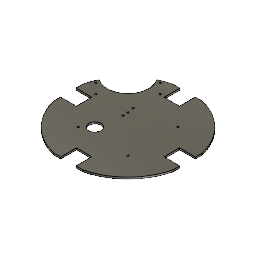
Rambots v6 (Autodesk Fusion 360 design; units mm, degrees)
Autodesk Fusion 360 part; units mm, degrees
sketch "Sketch2" plane through (0, 0, 0) normal (0, 0, 1) x (1, 0, 0) in component "Base plate"
  circle A0 centre (0, 0) radius 105
  line L0 (0, 0) -> (0, 105)
  line L1 (0, 0) -> (0, -105)
  line L2 (0, 0) -> (105, 0)
  line L3 (0, 0) -> (-105, 0)
  line L4 (-105, 0) -> (-102, 0)
  line L5 (-102, 0) -> (-102, 24.9199)
  line L6 (-102, 0) -> (-102, -24.9199)
  line L7 (-102, 24.9199) -> (-75, 24.9199)
  line L8 (-102, -24.9199) -> (-75, -24.9199)
  line L9 (-75, -24.9199) -> (-75, 24.9199)
  line L10 (0, 105) -> (0, 102)
  line L11 (0, 102) -> (24.9199, 102)
  line L12 (0, 102) -> (-24.9199, 102)
  line L13 (-24.9199, 102) -> (-24.9199, 75)
  line L14 (24.9199, 102) -> (24.9199, 75)
  line L15 (24.9199, 75) -> (-24.9199, 75)
  line L16 (105, 0) -> (102, 0)
  line L17 (102, 0) -> (102, 24.9199)
  line L18 (102, 0) -> (102, -24.9199)
  line L19 (102, -24.9199) -> (75, -24.9199)
  line L20 (102, 24.9199) -> (75, 24.9199)
  line L21 (75, 24.9199) -> (75, -24.9199)
  line L22 (0, -105) -> (0, -102)
  line L23 (0, -102) -> (24.9199, -102)
  line L24 (0, -102) -> (-24.9199, -102)
  line L25 (-24.9199, -102) -> (-24.9199, -75)
  line L26 (24.9199, -102) -> (24.9199, -75)
  line L27 (24.9199, -75) -> (-24.9199, -75)
  line L28 (0, 0) -> (3.7123, -3.7123)
  line L29 (0, 0) -> (5.25, 0) construction
  line L30 (0, 0) -> (-3.7123, 3.7123)
  line L31 (0, 0) -> (5.25, 0) construction
  line L32 (-3.7123, 3.7123) -> (-1.591, 5.8336)
  line L33 (-1.591, 5.8336) -> (8.909, 5.8336) construction
  line L34 (5.8336, -1.591) -> (3.7123, -3.7123)
  line L35 (3.7123, -3.7123) -> (1.591, -5.8336)
  line L36 (3.7123, -3.7123) -> (6.7123, -3.7123) construction
  line L37 (1.591, -5.8336) -> (12.091, -5.8336) construction
  line L38 (-5.8336, 1.591) -> (-3.7123, 3.7123)
  line L39 (-3.7123, 3.7123) -> (-1.591, 5.8336)
  line L40 (-75, 0) -> (-67.5, 0)
  line L41 (-67.5, 0) -> (-67.5, 13)
  line L42 (-67.5, 13) -> (-75, 13)
  line L43 (-75, 13) -> (-75, 0)
  line L44 (-67.5, 0) -> (-75, 0)
  line L45 (-75, 0) -> (-75, -13)
  line L46 (-75, -13) -> (-67.5, -13)
  line L47 (-67.5, -13) -> (-67.5, 0)
  line L48 (0, 75) -> (-13, 75)
  line L49 (-13, 75) -> (-13, 67.5)
  line L50 (-13, 67.5) -> (0, 67.5)
  line L51 (0, 67.5) -> (0, 75)
  line L52 (10, 75) -> (0, 75)
  line L53 (0, 75) -> (0, 67.5)
  line L54 (75, 0) -> (67.5, 0)
  line L55 (67.5, 0) -> (67.5, 13)
  line L56 (67.5, 13) -> (75, 13)
  line L57 (75, 13) -> (75, 0)
  line L58 (67.5, 0) -> (75, 0)
  line L59 (75, 0) -> (75, -10)
  line L60 (0, -75) -> (13, -75)
  line L61 (13, -75) -> (13, -67.5)
  line L62 (13, -67.5) -> (0, -67.5)
  line L63 (0, -67.5) -> (0, -75)
  line L64 (-10, -75) -> (0, -75)
  line L65 (0, -75) -> (0, -67.5)
  line L66 (0, -67.5) -> (-13, -67.5)
  line L67 (-13, -67.5) -> (-13, -75)
  line L68 (67.5, 0) -> (67.5, -13)
  line L69 (67.5, -13) -> (75, -13)
  line L70 (0, 67.5) -> (13, 67.5)
  line L71 (13, 67.5) -> (13, 75)
  line L72 (-13, 75) -> (-13, 102)
  line L73 (13, 75) -> (13, 102)
  line L74 (75, 13) -> (102, 13)
  line L75 (75, -13) -> (102, -13)
  line L76 (13, -75) -> (13, -102)
  line L77 (-13, -75) -> (-13, -102)
  line L78 (-75, -13) -> (-102, -13)
  line L79 (-75, 13) -> (-102, 13)
  dimension "d2" = 210
  dimension "d3" = 3
  dimension "d4" = 27
  dimension "d5" = 27
  dimension "d6" = 3
  dimension "d7" = 27
  dimension "d8" = 27
  dimension "d9" = 3
  dimension "d10" = 27
  dimension "d11" = 27
  dimension "d12" = 3
  dimension "d13" = 27
  dimension "d14" = 27
  dimension "d15" = 45
  dimension "d16" = 5.25
  dimension "d17" = 135
  dimension "d18" = 5.25
  dimension "d19" = 3
  dimension "d21" = 10.5
  dimension "d22" = 135
  dimension "d23" = 3
  dimension "d25" = 10.5
  dimension "d28" = 7.5
  dimension "d29" = 13
  dimension "d30" = 13
  dimension "d31" = 7.5
  dimension "d32" = 7.5
  dimension "d33" = 13
  dimension "d34" = 7.5
  dimension "d35" = 13
  dimension "d36" = 7.5
  dimension "d37" = 13
  dimension "d96" = 13
  dimension "d97" = 13
  dimension "d98" = 13
  dimension "d99" = 27
  constraint coincident A0.centre L0.start
  constraint coincident A0 L0.end
  constraint vertical L0
  constraint coincident A0 L1.end
  constraint parallel L0 L1
  constraint coincident A0 L2.end
  constraint perpendicular L1 L2
  constraint coincident A0 L3.end
  constraint perpendicular L1 L3
  constraint parallel L3 L4
  constraint vertical L5
  constraint coincident A0 L5.end
  constraint vertical L6
  constraint coincident A0 L6.end
  constraint perpendicular L5 L7
  constraint perpendicular L6 L8
  constraint parallel L0 L10
  constraint horizontal L11
  constraint coincident A0 L11.end
  constraint horizontal L12
  constraint coincident A0 L12.end
  constraint perpendicular L12 L13
  constraint perpendicular L11 L14
  constraint horizontal L16
  constraint vertical L17
  constraint coincident A0 L17.end
  constraint vertical L18
  constraint coincident A0 L18.end
  constraint perpendicular L18 L19
  constraint horizontal L20
  constraint perpendicular L19 L22
  constraint horizontal L23
  constraint coincident A0 L23.end
  constraint coincident A0 L24.end
  constraint perpendicular L1 L24
  constraint perpendicular L24 L25
  constraint vertical L26
  constraint horizontal L29
  constraint horizontal L31
  constraint perpendicular L30 L32
  constraint horizontal L33
  constraint horizontal L36
  constraint horizontal L37
  constraint horizontal L40
  constraint vertical L41
  constraint horizontal L42
  constraint vertical L43
  constraint midpoint L9 L40.start
  constraint horizontal L44
  constraint vertical L45
  constraint horizontal L46
  constraint vertical L47
  constraint horizontal L48
  constraint vertical L49
  constraint horizontal L50
  constraint vertical L51
  constraint midpoint L15 L48.start
  constraint horizontal L52
  constraint vertical L53
  constraint coincident L15 L52.start
  constraint horizontal L54
  constraint vertical L55
  constraint horizontal L56
  constraint vertical L57
  constraint midpoint L21 L54.start
  constraint horizontal L58
  constraint vertical L59
  constraint coincident L21 L59.end
  constraint horizontal L60
  constraint vertical L61
  constraint horizontal L62
  constraint vertical L63
  constraint midpoint L27 L60.start
  constraint horizontal L64
  constraint vertical L65
  constraint coincident L27 L64.start
  constraint perpendicular L1 L66
  constraint coincident L27 L67.end
  constraint perpendicular L27 L67
  constraint perpendicular L58 L68
  constraint coincident L21 L69.end
  constraint perpendicular L21 L69
  constraint perpendicular L51 L70
  constraint coincident L15 L71.end
  constraint perpendicular L15 L71
  constraint coincident L12 L72.end
  constraint perpendicular L12 L72
  constraint coincident L11 L73.end
  constraint perpendicular L11 L73
  constraint coincident L17 L74.end
  constraint perpendicular L17 L74
  constraint coincident L18 L75.end
  constraint perpendicular L18 L75
  constraint coincident L23 L76.end
  constraint perpendicular L23 L76
  constraint coincident L24 L77.end
  constraint perpendicular L24 L77
  constraint coincident L6 L78.end
  constraint perpendicular L6 L78
  constraint coincident L5 L79.end
  constraint perpendicular L5 L79
  measures "d2" diameter of A0
  measures "d3" distance of L3.end L4.end
  measures "d4" distance of L5.end L7.end
  measures "d5" distance of L6.end L8.end
  measures "d6" distance of L0.end L10.end
  measures "d7" distance of L12.end L13.end
  measures "d8" distance of L11.end L14.end
  measures "d9" distance of L2.end L16.end
  measures "d10" distance of L18.end L19.end
  measures "d11" distance of L17.end L20.end
  measures "d12" distance of L1.end L22.end
  measures "d13" distance of L24.end L25.end
  measures "d14" distance of L23.end L26.end
  measures "d15" angle of L28 L29
  measures "d16" distance of A0.centre L28.end
  measures "d17" angle of L30 L31
  measures "d18" distance of A0.centre L30.end
  measures "d19" distance of L30.end L32.end
  measures "d21" distance of L32.end L34.start
  measures "d22" angle of L35 L36
  measures "d23" distance of L28.end L35.end
  measures "d25" distance of L35.end L38.start
  measures "d28" distance of L40.start L40.end
  measures "d29" distance of L40.start L42.end
  measures "d30" distance of L40.end L46.end
  measures "d31" distance of L40.end L40.start
  measures "d32" distance of L48.start L50.end
  measures "d33" distance of L48.start L48.end
  measures "d34" distance of L54.start L54.end
  measures "d35" distance of L54.start L56.end
  measures "d36" distance of L60.start L62.end
  measures "d37" distance of L60.start L60.end
  measures "d96" distance of L62.end L66.end
  measures "d97" distance of L54.end L68.end
  measures "d98" distance of L50.end L70.end
  measures "d99" distance of L69.end L75.end
extrude "Extrude2" add sketch "Sketch2" along normal blind 3.175 contours A0 L0 L2 L14 L15 L20 L21 L55 L56 L70 L71 | L17 L20 L21 L74 | L18 L19 L21 L75 | A0 L1 L2 L19 L21 L26 L27 L61 L62 L68 L69 | L11 L14 L15 L73 | L23 L26 L27 L76 | L2 L21 L54 L58 L59 L68 L69 | L2 L21 L54 L55 L56 L57 L58 | A0 L0 L3 L7 L9 L13 L15 L41 L42 L49 L50 | L12 L13 L15 L72 | L0 L15 L51 L52 L53 L70 L71 | L24 L25 L27 L77 | A0 L1 L3 L8 L9 L25 L27 L46 L47 L66 L67 | L1 L27 L60 L61 L62 L63 L65 | L5 L7 L9 L79 | L0 L15 L48 L49 L50 L51 L53 | L6 L8 L9 L78 | L1 L27 L63 L64 L65 L66 L67 | L3 L9 L40 L44 L45 L46 L47 | L3 L9 L40 L41 L42 L43 L44 in component "Base plate"
sketch "Sketch3" plane through (0, 0, 0) normal (0, 0, -1) x (1, 0, 0) in component "Base plate"
  arc A0 (-102, -24.9199) -> (-24.9199, -102) centre (0, 0) ccw
  line L0 (13, 75) -> (-13, 75)
  line L1 (-75, 13) -> (-75, -13)
  line L2 (-13, -75) -> (13, -75)
  line L3 (75, -13) -> (75, 13)
  line L4 (-67.5, 0) -> (-65.5, 0)
  line L5 (-65.5, 0) -> (-24.25, 0)
  line L6 (-24.25, 0) -> (-24.25, 10)
  line L7 (-24.25, 10) -> (-65.5, 10)
  line L8 (-65.5, 10) -> (-65.5, 0)
  line L9 (-65.5, 0) -> (-24.25, 0)
  line L10 (-24.25, 0) -> (-24.25, -10)
  line L11 (-24.25, -10) -> (-65.5, -10)
  line L12 (-65.5, -10) -> (-65.5, 0)
  line L13 (-24.25, 0) -> (-11.25, 0)
  line L14 (-65.5, 0) -> (-59.5, 0)
  circle A1 centre (-59.5, 0) radius 1.5
  line L15 (-65.5, 10) -> (-57.75, 10)
  line L16 (-57.75, 10) -> (-56.25, 10)
  line L17 (-56.25, 10) -> (-56.25, 8)
  circle A2 centre (-56.25, 8) radius 1.5
  line L18 (-57.75, 10) -> (-57.75, 8)
  line L19 (-56.25, 10) -> (-54.75, 10)
  line L20 (-54.75, 10) -> (-54.75, 8)
  line L21 (-65.5, -10) -> (-57.75, -10)
  line L22 (-57.75, -10) -> (-56.25, -10)
  line L23 (-56.25, -10) -> (-54.75, -10)
  line L24 (-56.25, -10) -> (-56.25, -8)
  circle A3 centre (-56.25, -8) radius 1.5
  line L25 (-57.75, -10) -> (-57.75, -8)
  line L26 (-54.75, -10) -> (-54.75, -8)
  line L27 (-54.75, -10) -> (-32.4, -10)
  line L28 (-54.75, 10) -> (-32.4, 10)
  line L29 (-32.4, 10) -> (-30.9, 10)
  line L30 (-30.9, 10) -> (-29.4, 10)
  line L31 (-32.4, -10) -> (-30.9, -10)
  line L32 (-30.9, -10) -> (-29.4, -10)
  line L33 (-30.9, 10) -> (-30.9, 8)
  circle A4 centre (-30.9, 8) radius 1.5
  line L34 (-32.4, 10) -> (-32.4, 8)
  line L35 (-29.4, 10) -> (-29.4, 8)
  line L36 (-30.9, -10) -> (-30.9, -8)
  circle A5 centre (-30.9, -8) radius 1.5
  line L37 (-32.4, -10) -> (-32.4, -8)
  line L38 (-29.4, -10) -> (-29.4, -8)
  line L39 (2.1213, -2.1213) -> (14.4957, -14.4957)
  circle A6 centre (14.4957, -14.4957) radius 1.5
  line L40 (0, 0) -> (-74.2462, -74.2462)
  line L41 (-74.2462, -74.2462) -> (-56.5685, -56.5685)
  line L42 (0, 0) -> (-28.2843, 28.2843)
  line L43 (0, 0) -> (35, 0) construction
  circle A7 centre (-28.2843, 28.2843) radius 7.5
  line L44 (-102, 13) -> (-75, 13)
  line L45 (-75, -13) -> (-102, -13)
  line L46 (-102, -13) -> (-102, -24.9199)
  line L47 (-24.9199, -102) -> (-13, -102)
  line L48 (-13, -102) -> (-13, -75)
  line L49 (13, -75) -> (13, -102)
  line L50 (13, -102) -> (24.9199, -102)
  arc A8 (24.9199, -102) -> (102, -24.9199) centre (0, 0) ccw
  line L51 (102, -24.9199) -> (102, -13)
  line L52 (102, -13) -> (75, -13)
  line L53 (75, 13) -> (102, 13)
  line L54 (102, 13) -> (102, 24.9199)
  arc A9 (102, 24.9199) -> (24.9199, 102) centre (0, 0) ccw
  line L55 (24.9199, 102) -> (13, 102)
  line L56 (13, 102) -> (13, 75)
  line L57 (-13, 75) -> (-13, 102)
  line L58 (-13, 102) -> (-24.9199, 102)
  arc A10 (-24.9199, 102) -> (-102, 24.9199) centre (0, 0) ccw
  line L59 (-102, 24.9199) -> (-102, 13)
  circle A11 centre (-74.2462, -74.2462) radius 35
  line L60 (0, 0) -> (-21.2132, -21.2132)
  circle A12 centre (-21.2132, -21.2132) radius 1.5
  dimension "d40" = 2
  dimension "d41" = 41.25
  dimension "d42" = 10
  dimension "d43" = 10
  dimension "d44" = 41.25
  dimension "d45" = 13
  dimension "d46" = 6
  dimension "d47" = 3
  dimension "d48" = 7.75
  dimension "d49" = 1.5
  dimension "d50" = 3
  dimension "d51" = 1.5
  dimension "d52" = 7.75
  dimension "d53" = 1.5
  dimension "d54" = 1.5
  dimension "d55" = 2
  dimension "d56" = 3
  dimension "d57" = 22.35
  dimension "d58" = 22.35
  dimension "d59" = 1.5
  dimension "d60" = 1.5
  dimension "d61" = 1.5
  dimension "d62" = 1.5
  dimension "d63" = 2
  dimension "d64" = 3
  dimension "d65" = 2
  dimension "d66" = 3
  dimension "d67" = 2
  dimension "d72" = 17.5
  dimension "d73" = 3
  dimension "d77" = 25
  dimension "d90" = 135
  dimension "d91" = 40
  dimension "d93" = 15
  dimension "d105" = 70
  dimension "d106" = 30
  dimension "d107" = 3
  constraint horizontal L4
  constraint horizontal L5
  constraint vertical L6
  constraint horizontal L7
  constraint vertical L8
  constraint horizontal L9
  constraint vertical L10
  constraint horizontal L11
  constraint vertical L12
  constraint perpendicular L6 L13
  constraint perpendicular L8 L14
  constraint coincident L14.end A1.centre
  constraint perpendicular L8 L15
  constraint parallel L7 L16
  constraint perpendicular L16 L17
  constraint coincident L17.end A2.centre
  constraint coincident A2 L18.end
  constraint tangent A2 L18
  constraint perpendicular L7 L18
  constraint perpendicular L18 L19
  constraint coincident A2 L20.end
  constraint tangent A2 L20
  constraint perpendicular L19 L20
  constraint perpendicular L12 L21
  constraint parallel L11 L22
  constraint parallel L11 L23
  constraint perpendicular L23 L24
  constraint coincident L24.end A3.centre
  constraint coincident A3 L25.end
  constraint tangent A3 L25
  constraint coincident A3 L26.end
  constraint tangent A3 L26
  constraint perpendicular L26 L27
  constraint perpendicular L20 L28
  constraint parallel L7 L29
  constraint parallel L7 L30
  constraint parallel L11 L31
  constraint parallel L11 L32
  constraint perpendicular L29 L33
  constraint coincident L33.end A4.centre
  constraint coincident A4 L34.end
  constraint tangent A4 L34
  constraint coincident A4 L35.end
  constraint tangent A4 L35
  constraint perpendicular L32 L36
  constraint coincident L36.end A5.centre
  constraint coincident A5 L37.end
  constraint tangent A5 L37
  constraint coincident A5 L38.end
  constraint tangent A5 L38
  constraint coincident L39.end A6.centre
  constraint coincident A0.centre L40.start
  constraint parallel L40 L41
  constraint horizontal L43
  constraint coincident L42.end A7.centre
  constraint coincident L40.end L41.start
  constraint perpendicular L42 L60
  constraint coincident L60.end A12.centre
  measures "d40" distance of L4.start L4.end
  measures "d41" distance of L4.end L5.end
  measures "d42" distance of L4.end L7.end
  measures "d43" distance of L4.end L11.end
  measures "d44" distance of L4.end L5.end
  measures "d45" distance of L5.end L13.end
  measures "d46" distance of L4.end L14.end
  measures "d47" diameter of A1
  measures "d48" distance of L7.end L15.end
  measures "d49" distance of L15.end L16.end
  measures "d50" diameter of A2
  measures "d51" distance of L16.end L19.end
  measures "d52" distance of L11.end L21.end
  measures "d53" distance of L21.end L22.end
  measures "d54" distance of L22.end L23.end
  measures "d55" distance of L22.end L24.end
  measures "d56" diameter of A3
  measures "d57" distance of L23.end L27.end
  measures "d58" distance of L19.end L28.end
  measures "d59" distance of L28.end L29.end
  measures "d60" distance of L29.end L30.end
  measures "d61" distance of L27.end L31.end
  measures "d62" distance of L31.end L32.end
  measures "d63" distance of L29.end L33.end
  measures "d64" diameter of A4
  measures "d65" distance of L31.end L36.end
  measures "d66" diameter of A5
  measures "d67" distance of L16.end L17.end
  measures "d72" distance of L39.start L39.end
  measures "d73" diameter of A6
  measures "d77" distance of L40.end L41.end
  measures "d90" angle of L42 L43
  measures "d91" distance of A0.centre L42.end
  measures "d93" diameter of A7
  measures "d105" diameter of A11
  measures "d106" distance of A0.centre L60.end
  measures "d107" diameter of A12
sketch "Sketch1" plane through (0, 0, 0) normal (1, 0, 0) x (0, 1, 0) in component "Base plate"
  line L0 (-5.8336, 3.175) -> (1.591, 3.175)
  line L1 (0, 10) -> (0, -5)
  constraint perpendicular L0 L1
extrude "Extrude3" cut sketch "Sketch3" against normal blind 20 contours A0 L40 L41 A11 | A0 L40 L41 A11 in component "Base plate"
sketch "Sketch2 (1)" plane through (0, 0, 3.175) normal (0, 0, 1) x (-1, 0, 0) in component "Base plate"
  line L0 (75, -13) -> (75, 13)
  line L1 (13, 75) -> (-13, 75)
  arc A0 (94.524, -45.7188) -> (102, -24.9199) centre (0, 0) ccw
  line L2 (-75, 13) -> (-75, -13)
  line L3 (-13, -75) -> (13, -75)
  line L4 (0, 0) -> (-42.4264, -42.4264)
  line L5 (0, 0) -> (65, 0) construction
  line L6 (-15.5563, -15.5563) -> (-33.9411, -33.9411)
  circle A1 centre (-42.4264, -42.4264) radius 1.5
  line L7 (102, -24.9199) -> (102, -13)
  line L8 (102, -13) -> (75, -13)
  line L9 (75, 13) -> (102, 13)
  line L10 (102, 13) -> (102, 24.9199)
  arc A2 (102, 24.9199) -> (24.9199, 102) centre (0, 0) ccw
  line L11 (24.9199, 102) -> (13, 102)
  line L12 (13, 102) -> (13, 75)
  line L13 (-13, 75) -> (-13, 102)
  line L14 (-13, 102) -> (-24.9199, 102)
  arc A3 (-24.9199, 102) -> (-102, 24.9199) centre (0, 0) ccw
  line L15 (-102, 24.9199) -> (-102, 13)
  line L16 (-102, 13) -> (-75, 13)
  line L17 (-75, -13) -> (-102, -13)
  line L18 (-102, -13) -> (-102, -24.9199)
  arc A4 (-102, -24.9199) -> (-24.9199, -102) centre (0, 0) ccw
  line L19 (-24.9199, -102) -> (-13, -102)
  line L20 (-13, -102) -> (-13, -75)
  line L21 (13, -75) -> (13, -102)
  line L22 (13, -102) -> (24.9199, -102)
  arc A5 (24.9199, -102) -> (45.7188, -94.524) centre (0, 0) ccw
  arc A6 (94.524, -45.7188) -> (45.7188, -94.524) centre (74.2462, -74.2462) ccw
  dimension "d82" = 135
  dimension "d83" = 60
  dimension "d84" = 26
  dimension "d85" = 3
  constraint horizontal L5
  constraint coincident A0.centre L4.start
  constraint coincident L4 L6.start
  constraint parallel L4 L6
  constraint coincident L4.end A1.centre
  measures "d82" angle of L4 L5
  measures "d83" distance of A0.centre L4.end
  measures "d84" distance of L6.start L6.end
  measures "d85" diameter of A1
extrude "Extrude4" cut sketch "Sketch2 (1)" against normal blind 10 contours A1 in component "Base plate"
pattern_circular "C-Pattern2" count 4 over 360 about axis through (0, 0, 1.75) along (0, 0, 1) of 1 faces at (43.8086, 41.8438, 2.1167) in component "Base plate"
extrude "Extrude5" cut sketch "Sketch3" against normal blind 20 contours A7 in component "Base plate"
sketch "Sketch4" plane through (0, 0, 0) normal (1, 0, 0) x (0, 1, 0)
sketch "Sketch5" plane through (0, 0, 3.175) normal (0, 0, 1) x (-1, 0, 0)
  circle A0 centre (28.2843, 28.2843) radius 7.5
  circle A1 centre (-42.4264, 42.4264) radius 1.5
  circle A2 centre (42.4264, 42.4264) radius 1.5
  circle A3 centre (42.4264, -42.4264) radius 1.5
  circle A4 centre (-42.4264, -42.4264) radius 1.5
  arc A5 (94.524, -45.7188) -> (102, -24.9199) centre (0, 0) ccw
  line L0 (102, -24.9199) -> (102, -13)
  line L1 (102, -13) -> (75, -13)
  line L2 (75, -13) -> (75, 13)
  line L3 (75, 13) -> (102, 13)
  line L4 (102, 13) -> (102, 24.9199)
  arc A6 (102, 24.9199) -> (24.9199, 102) centre (0, 0) ccw
  line L5 (24.9199, 102) -> (13, 102)
  line L6 (13, 102) -> (13, 75)
  line L7 (13, 75) -> (-13, 75)
  line L8 (-13, 75) -> (-13, 102)
  line L9 (-13, 102) -> (-24.9199, 102)
  arc A7 (-24.9199, 102) -> (-102, 24.9199) centre (0, 0) ccw
  line L10 (-102, 24.9199) -> (-102, 13)
  line L11 (-102, 13) -> (-75, 13)
  line L12 (-75, 13) -> (-75, -13)
  line L13 (-75, -13) -> (-102, -13)
  line L14 (-102, -13) -> (-102, -24.9199)
  arc A8 (-102, -24.9199) -> (-24.9199, -102) centre (0, 0) ccw
  line L15 (-24.9199, -102) -> (-13, -102)
  line L16 (-13, -102) -> (-13, -75)
  line L17 (-13, -75) -> (13, -75)
  line L18 (13, -75) -> (13, -102)
  line L19 (13, -102) -> (24.9199, -102)
  arc A9 (24.9199, -102) -> (45.7188, -94.524) centre (0, 0) ccw
  line L20 (0, 0) -> (-21.2132, -21.2132)
  line L21 (0, 0) -> (30, 0) construction
  circle A10 centre (-21.2132, -21.2132) radius 1.5
  arc A11 (94.524, -45.7188) -> (45.7188, -94.524) centre (74.2462, -74.2462) ccw
  dimension "d100" = 135
  dimension "d101" = 30
  dimension "d102" = 3
  constraint horizontal L21
  constraint coincident A5.centre A6.centre
  constraint coincident L20.end A10.centre
  measures "d100" angle of L20 L21
  measures "d101" distance of A5.centre L20.end
  measures "d102" diameter of A10
extrude "Extrude6" cut sketch "Sketch5" against normal blind 35 contours A10 in component "Base plate"
extrude "Extrude7" cut sketch "Sketch3" against normal blind 6 contours L40 L60 A12 | L40 L60 A12 in component "Base plate"
sketch "Sketch6" plane through (0, 0, 3.175) normal (0, 0, 1) x (-1, 0, 0)
  circle A0 centre (21.2132, -21.2132) radius 1.5
  circle A1 centre (-21.2132, -21.2132) radius 1.5
  circle A2 centre (28.2843, 28.2843) radius 7.5
  circle A3 centre (-42.4264, 42.4264) radius 1.5
  circle A4 centre (42.4264, 42.4264) radius 1.5
  circle A5 centre (42.4264, -42.4264) radius 1.5
  circle A6 centre (-42.4264, -42.4264) radius 1.5
  arc A7 (94.524, -45.7188) -> (45.7188, -94.524) centre (74.2462, -74.2462) ccw
  arc A8 (94.524, -45.7188) -> (102, -24.9199) centre (0, 0) ccw
  line L0 (102, -24.9199) -> (102, -13)
  line L1 (102, -13) -> (75, -13)
  line L2 (75, -13) -> (75, 13)
  line L3 (75, 13) -> (102, 13)
  line L4 (102, 13) -> (102, 24.9199)
  arc A9 (102, 24.9199) -> (24.9199, 102) centre (0, 0) ccw
  line L5 (24.9199, 102) -> (13, 102)
  line L6 (13, 102) -> (13, 75)
  line L7 (13, 75) -> (-13, 75)
  line L8 (-13, 75) -> (-13, 102)
  line L9 (-13, 102) -> (-24.9199, 102)
  arc A10 (-24.9199, 102) -> (-102, 24.9199) centre (0, 0) ccw
  line L10 (-102, 24.9199) -> (-102, 13)
  line L11 (-102, 13) -> (-75, 13)
  line L12 (-75, 13) -> (-75, -13)
  line L13 (-75, -13) -> (-102, -13)
  line L14 (-102, -13) -> (-102, -24.9199)
  arc A11 (-102, -24.9199) -> (-24.9199, -102) centre (0, 0) ccw
  line L15 (-24.9199, -102) -> (-13, -102)
  line L16 (-13, -102) -> (-13, -75)
  line L17 (-13, -75) -> (13, -75)
  line L18 (13, -75) -> (13, -102)
  line L19 (13, -102) -> (24.9199, -102)
  arc A12 (24.9199, -102) -> (45.7188, -94.524) centre (0, 0) ccw
  circle A13 centre (42.4264, -42.4264) radius 1.5
  constraint concentric A5 A13
extrude "Extrude8" add sketch "Sketch6" against normal blind 3.175 contours A5 A13 in component "Base plate"
sketch "Sketch7" plane through (0, 0, 3.175) normal (0, 0, 1) x (-1, 0, 0)
  circle A0 centre (21.2132, -21.2132) radius 1.5
  circle A1 centre (-21.2132, -21.2132) radius 1.5
  circle A2 centre (28.2843, 28.2843) radius 7.5
  circle A3 centre (-42.4264, 42.4264) radius 1.5
  circle A4 centre (42.4264, 42.4264) radius 1.5
  circle A5 centre (-42.4264, -42.4264) radius 1.5
  arc A6 (94.524, -45.7188) -> (45.7188, -94.524) centre (74.2462, -74.2462) ccw
  arc A7 (94.524, -45.7188) -> (102, -24.9199) centre (0, 0) ccw
  line L0 (102, -24.9199) -> (102, -13)
  line L1 (102, -13) -> (75, -13)
  line L2 (75, -13) -> (75, 13)
  line L3 (75, 13) -> (102, 13)
  line L4 (102, 13) -> (102, 24.9199)
  arc A8 (102, 24.9199) -> (24.9199, 102) centre (0, 0) ccw
  line L5 (24.9199, 102) -> (13, 102)
  line L6 (13, 102) -> (13, 75)
  line L7 (13, 75) -> (-13, 75)
  line L8 (-13, 75) -> (-13, 102)
  line L9 (-13, 102) -> (-24.9199, 102)
  arc A9 (-24.9199, 102) -> (-102, 24.9199) centre (0, 0) ccw
  line L10 (-102, 24.9199) -> (-102, 13)
  line L11 (-102, 13) -> (-75, 13)
  line L12 (-75, 13) -> (-75, -13)
  line L13 (-75, -13) -> (-102, -13)
  line L14 (-102, -13) -> (-102, -24.9199)
  arc A10 (-102, -24.9199) -> (-24.9199, -102) centre (0, 0) ccw
  line L15 (-24.9199, -102) -> (-13, -102)
  line L16 (-13, -102) -> (-13, -75)
  line L17 (-13, -75) -> (13, -75)
  line L18 (13, -75) -> (13, -102)
  line L19 (13, -102) -> (24.9199, -102)
  arc A11 (24.9199, -102) -> (45.7188, -94.524) centre (0, 0) ccw
  circle A12 centre (28.2843, 28.2843) radius 10.5
  dimension "d112" = 21
  constraint concentric A2 A12
  measures "d112" diameter of A12
extrude "Extrude9" cut sketch "Sketch7" against normal blind 20 contours A12 in component "Base plate"
sketch "Sketch8" plane through (0, 0, 3.175) normal (0, 0, 1) x (-1, 0, 0)
  circle A0 centre (28.2843, 28.2843) radius 10.5
  circle A1 centre (21.2132, -21.2132) radius 1.5
  circle A2 centre (-21.2132, -21.2132) radius 1.5
  circle A3 centre (-42.4264, 42.4264) radius 1.5
  circle A4 centre (42.4264, 42.4264) radius 1.5
  circle A5 centre (-42.4264, -42.4264) radius 1.5
  arc A6 (94.524, -45.7188) -> (45.7188, -94.524) centre (74.2462, -74.2462) ccw
  arc A7 (94.524, -45.7188) -> (102, -24.9199) centre (0, 0) ccw
  line L0 (102, -24.9199) -> (102, -13)
  line L1 (102, -13) -> (75, -13)
  line L2 (75, -13) -> (75, 13)
  line L3 (75, 13) -> (102, 13)
  line L4 (102, 13) -> (102, 24.9199)
  arc A8 (102, 24.9199) -> (24.9199, 102) centre (0, 0) ccw
  line L5 (24.9199, 102) -> (13, 102)
  line L6 (13, 102) -> (13, 75)
  line L7 (13, 75) -> (-13, 75)
  line L8 (-13, 75) -> (-13, 102)
  line L9 (-13, 102) -> (-24.9199, 102)
  arc A9 (-24.9199, 102) -> (-102, 24.9199) centre (0, 0) ccw
  line L10 (-102, 24.9199) -> (-102, 13)
  line L11 (-102, 13) -> (-75, 13)
  line L12 (-75, 13) -> (-75, -13)
  line L13 (-75, -13) -> (-102, -13)
  line L14 (-102, -13) -> (-102, -24.9199)
  arc A10 (-102, -24.9199) -> (-24.9199, -102) centre (0, 0) ccw
  line L15 (-24.9199, -102) -> (-13, -102)
  line L16 (-13, -102) -> (-13, -75)
  line L17 (-13, -75) -> (13, -75)
  line L18 (13, -75) -> (13, -102)
  line L19 (13, -102) -> (24.9199, -102)
  arc A11 (24.9199, -102) -> (45.7188, -94.524) centre (0, 0) ccw
  circle A12 centre (-21.2132, -21.2132) radius 1.5
  constraint concentric A2 A12
extrude "Extrude10" add sketch "Sketch8" against normal blind 3.175 contours A2 A12 in component "Base plate"
sketch "Sketch9" plane through (0, 0, 0) normal (0, 0, -1) x (1, 0, 0)
  circle A0 centre (-28.2843, 28.2843) radius 10.5
  circle A1 centre (-21.2132, -21.2132) radius 1.5
  circle A2 centre (42.4264, 42.4264) radius 1.5
  circle A3 centre (-42.4264, 42.4264) radius 1.5
  circle A4 centre (42.4264, -42.4264) radius 1.5
  arc A5 (-45.7188, -94.524) -> (-94.524, -45.7188) centre (-74.2462, -74.2462) ccw
  arc A6 (-45.7188, -94.524) -> (-24.9199, -102) centre (0, 0) ccw
  line L0 (-24.9199, -102) -> (-13, -102)
  line L1 (-13, -102) -> (-13, -75)
  line L2 (-13, -75) -> (13, -75)
  line L3 (13, -75) -> (13, -102)
  line L4 (13, -102) -> (24.9199, -102)
  arc A7 (24.9199, -102) -> (102, -24.9199) centre (0, 0) ccw
  line L5 (102, -24.9199) -> (102, -13)
  line L6 (102, -13) -> (75, -13)
  line L7 (75, -13) -> (75, 13)
  line L8 (75, 13) -> (102, 13)
  line L9 (102, 13) -> (102, 24.9199)
  arc A8 (102, 24.9199) -> (24.9199, 102) centre (0, 0) ccw
  line L10 (24.9199, 102) -> (13, 102)
  line L11 (13, 102) -> (13, 75)
  line L12 (13, 75) -> (-13, 75)
  line L13 (-13, 75) -> (-13, 102)
  line L14 (-13, 102) -> (-24.9199, 102)
  arc A9 (-24.9199, 102) -> (-102, 24.9199) centre (0, 0) ccw
  line L15 (-102, 24.9199) -> (-102, 13)
  line L16 (-102, 13) -> (-75, 13)
  line L17 (-75, 13) -> (-75, -13)
  line L18 (-75, -13) -> (-102, -13)
  line L19 (-102, -13) -> (-102, -24.9199)
  arc A10 (-102, -24.9199) -> (-94.524, -45.7188) centre (0, 0) ccw
  line L20 (13, -75) -> (-75, 13)
  line L21 (-31, -31) -> (-23.2218, -38.7782)
  line L22 (-31, -31) -> (-38.7782, -23.2218)
  line L23 (-38.7782, -23.2218) -> (-35.2426, -19.6863)
  line L24 (-35.2426, -19.6863) -> (-19.6863, -35.2426)
  line L25 (-19.6863, -35.2426) -> (-23.2218, -38.7782)
  line L26 (-27.4645, -27.4645) -> (-23.2218, -31.7071)
  line L27 (-27.4645, -27.4645) -> (-31.7071, -23.2218)
  circle A11 centre (-23.2218, -31.7071) radius 1.5
  line L28 (-23.2218, -31.7071) -> (-12.6152, -21.1005)
  line L29 (-12.6152, -21.1005) -> (-21.1005, -12.6152)
  circle A12 centre (-21.1005, -12.6152) radius 1.5
  dimension "d117" = 11
  dimension "d118" = 11
  dimension "d119" = 5
  dimension "d120" = 22
  dimension "d121" = 6
  dimension "d122" = 6
  dimension "d123" = 3
  dimension "d124" = 15
  dimension "d125" = 12
  dimension "d126" = 3
  constraint coincident L2.end L3.start
  constraint coincident L16.end L17.start
  constraint midpoint L20 L21.start
  constraint parallel L20 L21
  constraint parallel L20 L22
  constraint perpendicular L22 L23
  constraint perpendicular L23 L24
  constraint midpoint L24 L26.start
  constraint perpendicular L25 L26
  constraint parallel L24 L27
  constraint coincident L26.end A11.centre
  constraint perpendicular L24 L28
  constraint perpendicular L28 L29
  constraint coincident L29.end A12.centre
  measures "d117" distance of L21.start L21.end
  measures "d118" distance of L21.start L22.end
  measures "d119" distance of L22.end L23.end
  measures "d120" distance of L23.end L24.end
  measures "d121" distance of L26.start L26.end
  measures "d122" distance of L26.start L27.end
  measures "d123" diameter of A11
  measures "d124" distance of L26.end L28.end
  measures "d125" distance of L28.end L29.end
  measures "d126" diameter of A12
extrude "Extrude11" cut sketch "Sketch9" against normal blind 16 contours L24 L26 A11 | L24 A11 L28 | L24 L26 A11 L28 | A12 in component "Base plate"
sketch "Sketch10" plane through (0, 0, 0) normal (0, 0, -1) x (1, 0, 0)
  circle A0 centre (-23.2218, -31.7071) radius 1.5
  circle A1 centre (-21.1005, -12.6152) radius 1.5
  circle A2 centre (-28.2843, 28.2843) radius 10.5
  circle A3 centre (-21.2132, -21.2132) radius 1.5
  circle A4 centre (42.4264, 42.4264) radius 1.5
  circle A5 centre (-42.4264, 42.4264) radius 1.5
  circle A6 centre (42.4264, -42.4264) radius 1.5
  arc A7 (-45.7188, -94.524) -> (-94.524, -45.7188) centre (-74.2462, -74.2462) ccw
  arc A8 (-45.7188, -94.524) -> (-24.9199, -102) centre (0, 0) ccw
  line L0 (-24.9199, -102) -> (-13, -102)
  line L1 (-13, -102) -> (-13, -75)
  line L2 (-13, -75) -> (13, -75)
  line L3 (13, -75) -> (13, -102)
  line L4 (13, -102) -> (24.9199, -102)
  arc A9 (24.9199, -102) -> (102, -24.9199) centre (0, 0) ccw
  line L5 (102, -24.9199) -> (102, -13)
  line L6 (102, -13) -> (75, -13)
  line L7 (75, -13) -> (75, 13)
  line L8 (75, 13) -> (102, 13)
  line L9 (102, 13) -> (102, 24.9199)
  arc A10 (102, 24.9199) -> (24.9199, 102) centre (0, 0) ccw
  line L10 (24.9199, 102) -> (13, 102)
  line L11 (13, 102) -> (13, 75)
  line L12 (13, 75) -> (-13, 75)
  line L13 (-13, 75) -> (-13, 102)
  line L14 (-13, 102) -> (-24.9199, 102)
  arc A11 (-24.9199, 102) -> (-102, 24.9199) centre (0, 0) ccw
  line L15 (-102, 24.9199) -> (-102, 13)
  line L16 (-102, 13) -> (-75, 13)
  line L17 (-75, 13) -> (-75, -13)
  line L18 (-75, -13) -> (-102, -13)
  line L19 (-102, -13) -> (-102, -24.9199)
  arc A12 (-102, -24.9199) -> (-94.524, -45.7188) centre (0, 0) ccw
  line L20 (-12.9026, -74.9862) -> (-31.2156, -56.6731)
  line L21 (-31.2156, -56.6731) -> (-40.2571, -65.7146)
  arc A13 (-40.2571, -65.7146) -> (-45.6948, -94.554) centre (-74.2861, -74.2307) cw
  arc A14 (-36.42, -98.5036) -> (-45.6948, -94.554) centre (0.1266, 0.182) cw
  line L22 (-36.42, -98.5036) -> (-12.9026, -74.9862)
  line L23 (-65.77, -40.2017) -> (-56.7285, -31.1602)
  line L24 (-56.7285, -31.1602) -> (-75.0416, -12.8472)
  line L25 (-75.0416, -12.8472) -> (-98.559, -36.3646)
  arc A15 (-94.6094, -45.6393) -> (-98.559, -36.3646) centre (0.1266, 0.182) cw
  arc A16 (-94.6094, -45.6394) -> (-65.77, -40.2017) centre (-74.2861, -74.2307) cw
  arc A17 (-19.9676, -76.9626) -> (-22.0937, -74.8366) centre (-21.0306, -75.8996) cw
  arc A18 (-22.0937, -74.8366) -> (-19.9676, -76.9626) centre (-21.0306, -75.8996) cw
  arc A19 (-36.8382, -93.8332) -> (-38.9643, -91.7072) centre (-37.9012, -92.7702) cw
  arc A20 (-38.9643, -91.7072) -> (-36.8382, -93.8332) centre (-37.9012, -92.7702) cw
  arc A21 (-93.8887, -36.7828) -> (-91.7626, -38.9089) centre (-92.8256, -37.8458) cw
  arc A22 (-91.7626, -38.9089) -> (-93.8887, -36.7828) centre (-92.8256, -37.8458) cw
  arc A23 (-77.018, -19.9122) -> (-74.892, -22.0382) centre (-75.955, -20.9752) cw
  arc A24 (-74.892, -22.0382) -> (-77.018, -19.9122) centre (-75.955, -20.9752) cw
extrude "Extrude12" cut sketch "Sketch10" against normal blind 17 contours A17 A18 | A19 A20 | A21 A22 | A23 A24 in component "Base plate"
component "Base plate" placed x (1, 0, 0) y (0, 1, 0) z (0, 0, 1) at (0, 0, 0)
